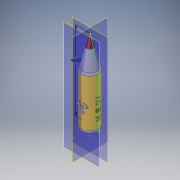
# Autodesk Inventor part: Pencil tooper
Saved by Autodesk Inventor 2018 (Build 220112000, 112)
## iProperties
Created: 2019-05-21
Part Number: Pencil tooper
Material: Generic
Document SubType Name: Modeling
Designer: 10043883
Density: 1 g/cm^3
Appearance: Default
Author: 10043883
Autodesk Inventor part; units mm, degrees
ref_plane "YZ Plane" through (0, 0, 0) normal (1, 0, 0) x (0, 1, 0)
sketch "Sketch1" plane through (0, 0, 0) normal (0, 0, 1) x (1, 0, 0)
  line L0 (0, 14.651) -> (23.1412, 14.651) construction
  line L1 (11.5706, 34.6919) -> (36.5111, 34.6919)
  line L2 (11.5706, 34.6919) -> (36.5111, 34.6919)
  line L3 (36.5111, 34.6919) -> (36.5111, 103.0971)
  line L4 (36.5111, 103.0971) -> (11.5706, 103.0971)
  line L5 (11.5706, 103.0971) -> (11.5706, 34.6919)
  line L6 (24.0409, 34.6919) -> (24.0409, 103.0971)
  line L7 (11.5706, 103.0971) -> (24.0409, 147.3983)
  line L8 (24.0409, 147.3983) -> (36.5111, 103.0971)
  line L9 (24.0409, 147.3983) -> (24.0409, 103.0971)
  line L10 (36.5111, 34.6919) -> (11.5706, 34.6919)
  line L11 (11.5706, 34.6919) -> (11.5706, 29.6166)
  line L12 (11.5706, 29.6166) -> (36.5111, 29.6166)
  line L13 (36.5111, 29.6166) -> (36.5111, 34.6919)
  line L14 (36.5111, 29.6166) -> (37.549, 25.9295)
  line L15 (37.549, 25.9295) -> (33.0115, 25.9295)
  line L16 (33.0115, 25.9295) -> (34.5814, 29.6166)
  line L17 (24.0409, 34.6919) -> (24.0409, 29.6166)
  point P0 (0, 0)
  point P1 (24.0409, 14.651)
  dimension "d29" = 117.7817
  constraints: 36 end point, 5 horizontal, 4 parallel, 3 midpoint, 2 perpendicular, 1 collinear, 1 point on line
  measures "d29" vertical distance of L7.end L11.end
sketch "Sketch2" plane through (0, 0, 0) normal (0, 0, 1) x (1, 0, 0)
  point P0 (0, 0)
revolve "Revolution2" add sketch "Sketch1" angle 360 about axis through (24.0409, 34.6919, 0) along (0, 1, 0) contours L5 L4 L6 L1
revolve "Revolution3" add sketch "Sketch1" angle 360 about axis through (24.0409, 147.3983, 0) along (0, -1, 0) contours L7 L9 L4
fillet "Fillet1" radius 201.6125 1 edges at (36.5111, 103.0971, 0)
ref_plane "Work Plane2" through (24.0409, 75.2622, 0) normal (0, 0, -1) x (0, 1, 0)
ref_plane "Work Plane3" through (24.0409, 75.2622, 0) normal (-1, 0, 0) x (0, 1, 0)
ref_plane "Work Plane4" through (24.0409, 75.2622, 0) normal (-0.7071068, 0, -0.7071068) x (0, 1, 0)
ref_plane "Work Plane5" through (11.5706, 68.8945, 0) normal (-1, 0, 0) x (0, -1, 0)
sketch "Sketch3" plane through (11.5706, 68.8945, 0) normal (-1, 0, 0) x (0, -1, 0)
  line L0 (-1.9865, 3.5619) -> (27.5239, 3.5619) construction
  line L1 (27.5239, 3.5619) -> (27.5239, 1.16) construction
  line L2 (27.5239, 1.16) -> (-1.9865, 1.16) construction
  line L3 (-1.9865, 1.16) -> (-1.9865, 3.5619) construction
  line L4 (-1.8911, -2.5341) -> (-2.2187, -2.5341)
  line L5 (-2.2187, -2.5341) -> (-2.2187, 3.5008)
  line L6 (-2.2187, 3.5008) -> (-1.8911, 3.5008)
  line L7 (-1.8911, 3.5008) -> (-1.8911, -2.5341)
  line L8 (1.0181, -2.1621) -> (0.5018, -2.6507)
  line L9 (0.5018, -2.6507) -> (-0.0201, -2.1621)
  line L10 (-0.0201, -2.1621) -> (0.5018, -1.6569)
  line L11 (0.5018, -1.6569) -> (1.0181, -2.1621)
  line L12 (0.5517, -2.1621) -> (0.5018, -2.1066)
  line L13 (0.5018, -2.1066) -> (0.4463, -2.1621)
  line L14 (0.4463, -2.1621) -> (0.5018, -2.2121)
  line L15 (0.5018, -2.2121) -> (0.5517, -2.1621)
  line L16 (7.2529, -1.0406) -> (6.9142, -1.7013)
  line L17 (6.9142, -1.7013) -> (6.3035, -2.2954)
  line L18 (6.3035, -2.2954) -> (5.6706, -2.5896)
  line L19 (5.6706, -2.5896) -> (4.4381, -2.5896)
  line L20 (4.4381, -2.5896) -> (3.8107, -2.2954)
  line L21 (3.8107, -2.2954) -> (3.1945, -1.7013)
  line L22 (3.1945, -1.7013) -> (2.9002, -1.1073)
  line L23 (2.9002, -1.1073) -> (2.5948, -0.2356)
  line L24 (2.5948, -0.2356) -> (2.5948, 1.1968)
  line L25 (2.5948, 1.1968) -> (2.9002, 2.0684)
  line L26 (2.9002, 2.0684) -> (3.1945, 2.6625)
  line L27 (3.1945, 2.6625) -> (3.8107, 3.2565)
  line L28 (3.8107, 3.2565) -> (4.4381, 3.5619)
  line L29 (4.4381, 3.5619) -> (5.6706, 3.5619)
  line L30 (5.6706, 3.5619) -> (6.3035, 3.2565)
  line L31 (6.3035, 3.2565) -> (6.9142, 2.6625)
  line L32 (6.9142, 2.6625) -> (7.2529, 2.0018)
  line L33 (7.2529, 2.0018) -> (6.9587, 1.8464)
  line L34 (6.9587, 1.8464) -> (6.6366, 2.4682)
  line L35 (6.6366, 2.4682) -> (6.0981, 2.99)
  line L36 (6.0981, 2.99) -> (5.5873, 3.2399)
  line L37 (5.5873, 3.2399) -> (4.5269, 3.2399)
  line L38 (4.5269, 3.2399) -> (4.0106, 2.99)
  line L39 (4.0106, 2.99) -> (3.4721, 2.4682)
  line L40 (3.4721, 2.4682) -> (3.1945, 1.9463)
  line L41 (3.1945, 1.9463) -> (2.928, 1.1524)
  line L42 (2.928, 1.1524) -> (2.928, -0.1912)
  line L43 (2.928, -0.1912) -> (3.1945, -0.9851)
  line L44 (3.1945, -0.9851) -> (3.4721, -1.507)
  line L45 (3.4721, -1.507) -> (4.0106, -2.0233)
  line L46 (4.0106, -2.0233) -> (4.5269, -2.2787)
  line L47 (4.5269, -2.2787) -> (5.5873, -2.2787)
  line L48 (5.5873, -2.2787) -> (6.0981, -2.0233)
  line L49 (6.0981, -2.0233) -> (6.6366, -1.507)
  line L50 (6.6366, -1.507) -> (6.9587, -0.8796)
  line L51 (6.9587, -0.8796) -> (7.2529, -1.0406)
  line L52 (10.9949, -2.1621) -> (10.4786, -2.6507)
  line L53 (10.4786, -2.6507) -> (9.9567, -2.1621)
  line L54 (9.9567, -2.1621) -> (10.4786, -1.6569)
  line L55 (10.4786, -1.6569) -> (10.9949, -2.1621)
  line L56 (10.5285, -2.1621) -> (10.4786, -2.1066)
  line L57 (10.4786, -2.1066) -> (10.423, -2.1621)
  line L58 (10.423, -2.1621) -> (10.4786, -2.2121)
  line L59 (10.4786, -2.2121) -> (10.5285, -2.1621)
  line L60 (17.2019, -1.3682) -> (16.891, -1.9789)
  line L61 (16.891, -1.9789) -> (16.5468, -2.3009)
  line L62 (16.5468, -2.3009) -> (15.6307, -2.5896)
  line L63 (15.6307, -2.5896) -> (12.8603, -2.5896)
  line L64 (12.8603, -2.5896) -> (12.8603, 3.5619)
  line L65 (12.8603, 3.5619) -> (15.6307, 3.5619)
  line L66 (15.6307, 3.5619) -> (16.5468, 3.2621)
  line L67 (16.5468, 3.2621) -> (16.891, 2.9456)
  line L68 (16.891, 2.9456) -> (17.2019, 2.3238)
  line L69 (17.2019, 2.3238) -> (17.2019, 1.6909)
  line L70 (17.2019, 1.6909) -> (16.891, 1.0746)
  line L71 (16.891, 1.0746) -> (16.5468, 0.7582)
  line L72 (16.5468, 0.7582) -> (16.1249, 0.6194)
  line L73 (16.1249, 0.6194) -> (16.5468, 0.4861)
  line L74 (16.5468, 0.4861) -> (16.891, 0.1641)
  line L75 (16.891, 0.1641) -> (17.2019, -0.4521)
  line L76 (17.2019, -0.4521) -> (17.2019, -1.3682)
  line L77 (16.8744, -1.2849) -> (16.8744, -0.5299)
  line L78 (16.8744, -0.5299) -> (16.6134, -0.0357)
  line L79 (16.6134, -0.0357) -> (16.3747, 0.203)
  line L80 (16.3747, 0.203) -> (15.5808, 0.4584)
  line L81 (15.5808, 0.4584) -> (13.1879, 0.4584)
  line L82 (13.1879, 0.4584) -> (13.1879, -2.2787)
  line L83 (13.1879, -2.2787) -> (15.5808, -2.2787)
  line L84 (15.5808, -2.2787) -> (16.3747, -2.0233)
  line L85 (16.3747, -2.0233) -> (16.6134, -1.7846)
  line L86 (16.6134, -1.7846) -> (16.8744, -1.2849)
  line L87 (16.8744, 1.7742) -> (16.8744, 2.2516)
  line L88 (16.8744, 2.2516) -> (16.6134, 2.7513)
  line L89 (16.6134, 2.7513) -> (16.3747, 2.9845)
  line L90 (16.3747, 2.9845) -> (15.5808, 3.2399)
  line L91 (15.5808, 3.2399) -> (13.1879, 3.2399)
  line L92 (13.1879, 3.2399) -> (13.1879, 0.7804)
  line L93 (13.1879, 0.7804) -> (15.5808, 0.7804)
  line L94 (15.5808, 0.7804) -> (16.3747, 1.0358)
  line L95 (16.3747, 1.0358) -> (16.6134, 1.2745)
  line L96 (16.6134, 1.2745) -> (16.8744, 1.7742)
  line L97 (20.9717, -2.1621) -> (20.4554, -2.6507)
  line L98 (20.4554, -2.6507) -> (19.9335, -2.1621)
  line L99 (19.9335, -2.1621) -> (20.4554, -1.6569)
  line L100 (20.4554, -1.6569) -> (20.9717, -2.1621)
  line L101 (20.5053, -2.1621) -> (20.4554, -2.1066)
  line L102 (20.4554, -2.1066) -> (20.3998, -2.1621)
  line L103 (20.3998, -2.1621) -> (20.4554, -2.2121)
  line L104 (20.4554, -2.2121) -> (20.5053, -2.1621)
  line L105 (27.7506, -2.5341) -> (27.423, -2.5341)
  line L106 (27.423, -2.5341) -> (27.423, 2.5348)
  line L107 (27.423, 2.5348) -> (25.4354, -2.5341)
  line L108 (25.4354, -2.5341) -> (25.1634, -2.5341)
  line L109 (25.1634, -2.5341) -> (23.1647, 2.5348)
  line L110 (23.1647, 2.5348) -> (23.1647, -2.5341)
  line L111 (23.1647, -2.5341) -> (22.8371, -2.5341)
  line L112 (22.8371, -2.5341) -> (22.8371, 3.5619)
  line L113 (22.8371, 3.5619) -> (23.1147, 3.5619)
  line L114 (23.1147, 3.5619) -> (25.2966, -1.9956)
  line L115 (25.2966, -1.9956) -> (27.4785, 3.5619)
  line L116 (27.4785, 3.5619) -> (27.7506, 3.5619)
  line L117 (27.7506, 3.5619) -> (27.7506, -2.5341)
  point P0 (68.8945, 0)
  constraints: 2 other
ref_plane "Work Plane6" through (24.0409, 68.8945, 12.4703) normal (0, 0, -1) x (-1, 0, 0)
sketch "Sketch4" plane through (24.0409, 68.8945, 12.4703) normal (0, 0, -1) x (-1, 0, 0)
  circle A0 centre (0, -11.126) radius 8.1934
  circle A1 centre (0, -11.126) radius 2.0662
  arc A2 (7.5469, -10.5193) -> (3.5904, -4.3922) centre (0.2113, -10.9152) ccw
  line L0 (3.6907, -4.4451) -> (1.3923, -8.8158)
  line L1 (7.5469, -10.5193) -> (2.7936, -10.9152)
  arc A3 (2.7936, -10.9152) -> (1.3923, -8.8158) centre (-0.2759, -11.4466) ccw
  arc A4 (-3.5951, -17.8314) -> (3.6981, -17.7535) centre (-0.0166, -11.4156) ccw
  line L2 (3.5998, -17.8101) -> (1.1291, -13.5344)
  line L3 (-3.5951, -17.8314) -> (-1.3941, -13.5997)
  arc A5 (-1.3941, -13.5997) -> (1.1291, -13.5344) centre (-0.2062, -10.72) ccw
  arc A6 (-3.0078, -4.2791) -> (-7.4254, -10.0827) centre (-0.1422, -11.0435) ccw
  line L4 (-7.4097, -9.9703) -> (-2.518, -10.6464)
  line L5 (-3.0078, -4.2791) -> (-1.0199, -8.615)
  arc A7 (-1.0199, -8.615) -> (-2.518, -10.6464) centre (0.5232, -11.3211) ccw
  point P0 (24.0409, -68.8945)
  constraints: 15 point on circle, 12 end point, 8 centre point, 1 coincident
extrude "Extrusion1" add sketch "Sketch4" along normal blind 25.4 contours A1 | L1 A3 L0 A2 | L3 A5 L2 A4 | L5 A7 L4 A6
extrude "Extrusion2" add sketch "Sketch3" against normal blind 25.4
revolve "Revolution4" add sketch "Sketch1" angle 360 about axis through (24.0409, 34.6919, 0) along (0, -1, 0) contours L6 L4 L3 L1 | L1 L13 L12 L17 | L14 L15 L16 L12
fillet "Fillet4" radius 3.175 2 edges at (11.5706, 103.0971, 0) (10.5327, 25.9295, 0)
body "Solid1"
